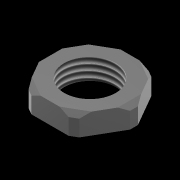
# Autodesk Inventor part: pg7_nut
Saved by Autodesk Inventor 2020.2 (Build 242310000, 310)
## iProperties
Created: 2020-04-23
Part Number: pg7_nut
Material: PC/ABS Plastic
Document SubType Name: Modeling
Designer: agmlego
Mass: 0.271981 g
Surface Area: 7.61813 cm^2
Volume: 0.761271 cm^3
Density: 0.357273 g/cm^3
Appearance: Smooth - Black
Author: agmlego
Autodesk Inventor part; units mm, degrees
ref_plane "YZ Plane" through (0, 0, 0) normal (1, 0, 0) x (0, 1, 0)
ref_plane "XZ Plane" through (0, 0, 0) normal (0, 1, 0) x (-1, 0, 0)
ref_plane "XY Plane" through (0, 0, 0) normal (0, 0, 1) x (1, 0, 0)
sketch "Sketch1" plane through (0, 0, 0) normal (0, 1, 0) x (-1, 0, 0)
  line L0 (10.248, 0) -> (5.124, -8.875)
  line L1 (5.124, -8.875) -> (-5.124, -8.875)
  line L2 (-5.124, -8.875) -> (-10.248, 0)
  line L3 (-10.248, 0) -> (-5.124, 8.875)
  line L4 (-5.124, 8.875) -> (5.124, 8.875)
  line L5 (5.124, 8.875) -> (10.248, 0)
  point P0 (0, 0)
  point P1 (0, 0)
  dimension "d0" = 17.75
  constraints: 12 end point, 1 coincident, 13 other
  measures "d0" distance between parallel lines of L1 L4
extrude "Extrusion1" add sketch "Sketch1" along normal blind 4.6
sketch "Sketch2" plane through (0, 4.6, 0) normal (0, 1, 0) x (1, 0, 0)
  point P0 (0, 0)
  point P1 (0, 0)
  constraints: 1 coincident
hole "Hole1" at (0, 4.6, 0) direction (0, -1, 0) diameter 11.445 end through all thread size "G13.157x1.337" designation "G 1/4" standard "DIN Pipe Threads"
chamfer "Chamfer1" distance 1 angle 45 6 edges at (5.124, 2.3, 8.875) (10.248, 2.3, 0) (5.124, 2.3, -8.875) (-5.124, 2.3, -8.875) (-10.248, 2.3, 0) (-5.124, 2.3, 8.875)
chamfer "Chamfer2" distance 1 angle 45 6 edges at (-4.874, 4.6, 8.442) (4.874, 4.6, 8.442) (9.748, 4.6, 0) (4.874, 4.6, -8.442) (-4.874, 4.6, -8.442) (-9.748, 4.6, 0)
body "Solid1"
